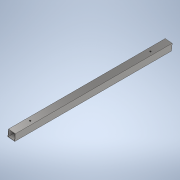
# Autodesk Inventor part: Asiento nuevo
Saved by Autodesk Inventor 2021 (Build 250183000, 183)
## iProperties
Created: 2014-11-01
Part Number: Asiento nuevo
Material: Acero, suave
Document SubType Name: Modeling
Designer: Yeison
Density: 7.85 g/cm^3
Appearance: Semipulido
Sending System: SolidWorks 2014
Last Author: JFGC
Last Saved: 2014-11-06
Author: Yeison
Autodesk Inventor part; units mm, degrees
ref_plane "YZ Plane" through (0, 0, 0) normal (1, 0, 0) x (0, 1, 0)
ref_plane "XZ Plane" through (0, 0, 0) normal (0, 1, 0) x (-1, 0, 0)
ref_plane "XY Plane" through (0, 0, 0) normal (0, 0, 1) x (1, 0, 0)
sketch "Boceto10" plane through (0, 0, 0) normal (0, 0, 1) x (1, 0, 0)
  line L0 (93.7879, -1.2643) -> (379.7634, -26.5882)
  line L1 (93.7879, -1.2643) -> (118.6905, -3.4695)
  line L2 (118.6905, -3.4695) -> (115.1622, -43.3135)
  line L3 (115.1622, -43.3135) -> (155.0063, -46.8418)
  line L4 (155.0063, -46.8418) -> (158.5346, -6.9978)
  line L5 (158.5346, -6.9978) -> (118.6905, -3.4695)
  line L6 (156.366, -8.8135) -> (153.1905, -44.6732)
  line L7 (153.1905, -44.6732) -> (117.3308, -41.4977)
  line L8 (117.3308, -41.4977) -> (120.5063, -5.6381)
  line L9 (120.5063, -5.6381) -> (156.366, -8.8135)
  line L10 (118.6905, -3.4695) -> (115.1622, -43.3135)
  line L11 (115.1622, -43.3135) -> (155.0063, -46.8418)
  line L12 (155.0063, -46.8418) -> (158.5346, -6.9978)
  line L13 (158.5346, -6.9978) -> (118.6905, -3.4695)
  point P0 (0, 0)
  dimension "d40" = 25
  dimension "l_c" = 40
  dimension "l_c2" = 40
  dimension "l_c3" = 40
  dimension "t_c" = 2
  constraints: 28 end point, 5 perpendicular, 2 parallel, 2 point on line, 3 other
  measures "d40" distance of L0.start L1.end
  measures "l_c" distance of L1.end L2.end
  measures "l_c2" distance of L2.end L3.end
  measures "l_c3" distance of L3.end L4.end
  measures "t_c" distance between parallel lines of L4 L6
extrude "Extrusión2" add sketch "Boceto10" against normal blind 900
sketch "Boceto12" plane through (158.5346, -6.9978, 0) normal (0.0882078, 0.9961021, 0) x (0.9961021, -0.0882078, 0)
  line L0 (-20.6136, 0) -> (-20.6136, 105)
  circle A0 centre (-20.6136, 105) radius 4
  line L1 (-38, 900) -> (-2, 900) projected
  line L2 (-20, 900) -> (-20, 795)
  circle A1 centre (-20, 795) radius 4
  point P0 (-158.5339, 0)
  dimension "d48" = 105
  dimension "d49" = 8
  dimension "d50" = 105
  dimension "d51" = 8
  constraints: 4 end point, 2 centre point, 2 coincident, 2 vertical, 1 midpoint
  measures "d48" distance of L0.start L0.end
  measures "d49" diameter of A0
  measures "d50" distance of L2.start L2.end
  measures "d51" diameter of A1
hole "Agujero1" at (138.0013, -5.1795, -105) at (138.6125, -5.2336, -795) direction (-0.0882078, -0.9961021, 0) diameter 8 end through all
equation "\"l_c2\" = l_c"
equation "\"l_c3\" = l_c"
